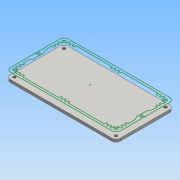
# Autodesk Inventor part: SZOMK-AK-C-C10-flat-plate
Saved by Autodesk Inventor 2016 (Build 200138000, 138)
## iProperties
Created: 2016-03-30
Part Number: SZOMK-AK-C-C10-flat-plate
Material: Generic
Document SubType Name: Modeling
Designer: admin
Density: 1 g/cm^3
Appearance: Default
Author: admin
Autodesk Inventor part; units mm, degrees
ref_plane "YZ Plane" through (0, 0, 0) normal (1, 0, 0) x (0, 1, 0)
ref_plane "XZ Plane" through (0, 0, 0) normal (0, 1, 0) x (-1, 0, 0)
ref_plane "XY Plane" through (0, 0, 0) normal (0, 0, 1) x (1, 0, 0)
derived "SZOMK-AK-C-C10-Walls.iam"
sketch "Sketch9" plane through (0, 0, 0) normal (0, 0, 1) x (1, 0, 0)
  line L0 (15.9674, 83.4048) -> (126.9674, 83.4048) projected
  arc A0 (15.9674, 83.4048) -> (11.4674, 78.9048) centre (15.9674, 78.9048) ccw projected
  line L1 (11.4674, 51.8798) -> (11.4674, 78.9048) projected
  line L2 (11.4674, 24.8548) -> (11.4674, 51.8798) projected
  arc A1 (11.4674, 24.8548) -> (15.9674, 20.3548) centre (15.9674, 24.8548) ccw projected
  line L3 (126.9674, 20.3548) -> (15.9674, 20.3548) projected
  arc A2 (126.9674, 20.3548) -> (131.4674, 24.8548) centre (126.9674, 24.8548) ccw projected
  line L4 (131.4674, 51.8798) -> (131.4674, 24.8548) projected
  line L5 (131.4674, 78.9048) -> (131.4674, 51.8798) projected
  arc A3 (131.4674, 78.9048) -> (126.9674, 83.4048) centre (126.9674, 78.9048) ccw projected
  point P0 (0, 0)
extrude "Extrusion3" add sketch "Sketch9" along normal blind 3
sketch "Sketch10" plane through (0, 0, 0) normal (0, 0, -1) x (-1, 0, 0)
  point P0 (0, 0)
  point P1 (-126.9674, 24.8548)
  point P2 (-126.9674, 78.9048)
  point P3 (-15.9674, 24.8548)
  point P4 (-15.9674, 78.9048)
hole "Hole1" at (126.9674, 78.9048, 0) at (126.9674, 24.8548, 0) at (15.9674, 24.8548, 0) at (15.9674, 78.9048, 0) direction (0, 0, 1) diameter 3 end through all countersink diameter 6 countersink angle 90
sketch "Sketch2" plane through (15.9674, 83.4048, 10) normal (0, 0, -1) x (1, 0, 0)
  line L0 (111, 31.525) -> (111, 24.3742) projected
  line L1 (111, 24.3742) -> (113, 21.6242) projected
  line L2 (113, 21.6242) -> (113, 15.7) projected
  line L3 (113, 15.7) -> (111, 15.7) projected
  line L4 (111, 15.7) -> (111, 13.7) projected
  line L5 (111, 13.7) -> (113, 13.7) projected
  line L6 (113, 13.7) -> (113, 11.7) projected
  line L7 (113, 11.7) -> (111, 11.7) projected
  line L8 (111, 11.7) -> (111, 9.7) projected
  line L9 (111, 9.7) -> (113, 9.7) projected
  line L10 (113, 9.7) -> (113, 7.3) projected
  line L11 (113, 7.3) -> (110.4678, 7.3) projected
  arc A0 (110.4678, 7.3) -> (110.1142, 6.4464) centre (110.4678, 6.8) ccw projected
  line L12 (110.1142, 6.4464) -> (110.6118, 5.9489) projected
  arc A1 (109.5511, 4.8882) -> (110.6118, 5.9489) centre (111, 4.5) ccw projected
  line L13 (109.5511, 4.8882) -> (109.0536, 5.3858) projected
  arc A2 (109.0536, 5.3858) -> (108.2, 5.0322) centre (108.7, 5.0322) ccw projected
  line L14 (108.2, 5.0322) -> (108.2, 2.3) projected
  line L15 (108.2, 2.3) -> (106.2, 2.3) projected
  line L16 (106.2, 2.3) -> (106.2, 4.5) projected
  line L17 (106.2, 4.5) -> (104.2, 4.5) projected
  line L18 (104.2, 4.5) -> (104.2, 2.3) projected
  line L19 (104.2, 2.3) -> (102.2, 2.3) projected
  line L20 (102.2, 2.3) -> (102.2, 4.5) projected
  line L21 (102.2, 4.5) -> (100.2, 4.5) projected
  line L22 (100.2, 4.5) -> (100.2, 2.3) projected
  line L23 (100.2, 2.3) -> (60.5, 2.3) projected
  line L24 (60.5, 2.3) -> (60.5, 4.5) projected
  line L25 (60.5, 4.5) -> (58.5, 4.5) projected
  line L26 (58.5, 4.5) -> (58.5, 2.3) projected
  line L27 (58.5, 2.3) -> (56.5, 2.3) projected
  line L28 (56.5, 2.3) -> (56.5, 4.5) projected
  line L29 (56.5, 4.5) -> (54.5, 4.5) projected
  line L30 (54.5, 4.5) -> (54.5, 2.3) projected
  line L31 (54.5, 2.3) -> (52.5, 2.3) projected
  line L32 (52.5, 2.3) -> (52.5, 4.5) projected
  line L33 (52.5, 4.5) -> (50.5, 4.5) projected
  line L34 (50.5, 4.5) -> (50.5, 2.3) projected
  line L35 (50.5, 2.3) -> (10.8, 2.3) projected
  line L36 (10.8, 2.3) -> (10.8, 4.5) projected
  line L37 (10.8, 4.5) -> (8.8, 4.5) projected
  line L38 (8.8, 4.5) -> (8.8, 2.3) projected
  line L39 (8.8, 2.3) -> (6.8, 2.3) projected
  line L40 (6.8, 2.3) -> (6.8, 4.5) projected
  line L41 (6.8, 4.5) -> (4.8, 4.5) projected
  line L42 (4.8, 4.5) -> (4.8, 2.3) projected
  line L43 (4.8, 2.3) -> (2.8, 2.3) projected
  line L44 (2.8, 2.3) -> (2.8, 5.0322) projected
  arc A3 (2.8, 5.0322) -> (1.9464, 5.3858) centre (2.3, 5.0322) ccw projected
  line L45 (1.9464, 5.3858) -> (1.4489, 4.8882) projected
  arc A4 (0.3882, 5.9489) -> (1.4489, 4.8882) centre (0, 4.5) ccw projected
  line L46 (0.3882, 5.9489) -> (0.8858, 6.4464) projected
  arc A5 (0.8858, 6.4464) -> (0.5322, 7.3) centre (0.5322, 6.8) ccw projected
  line L47 (0.5322, 7.3) -> (-2, 7.3) projected
  line L48 (-2, 7.3) -> (-2, 9.7) projected
  line L49 (-2, 9.7) -> (0, 9.7) projected
  line L50 (0, 9.7) -> (0, 11.7) projected
  line L51 (0, 11.7) -> (-2, 11.7) projected
  line L52 (-2, 11.7) -> (-2, 13.7) projected
  line L53 (-2, 13.7) -> (0, 13.7) projected
  line L54 (0, 13.7) -> (0, 15.7) projected
  line L55 (0, 15.7) -> (-2, 15.7) projected
  line L56 (-2, 15.7) -> (-2, 23.3362) projected
  line L57 (-2, 23.3362) -> (0, 26.7706) projected
  line L58 (0, 26.7706) -> (0, 31.525) projected
  line L59 (0, 31.525) -> (-1.5, 31.525) projected
  line L60 (-1.5, 31.525) -> (-1.5, 30.1864) projected
  arc A6 (-3, 30.1864) -> (-1.5, 30.1864) centre (-2.25, 29.525) ccw projected
  line L61 (-3, 30.1864) -> (-3, 31.525) projected
  line L62 (-3, 31.525) -> (-4.5, 31.525) projected
  line L63 (-4.5, 31.525) -> (-4.5, 4.5) projected
  arc A7 (-4.5, 4.5) -> (0, 0) centre (0, 4.5) ccw projected
  line L64 (0, 0) -> (111, 0) projected
  arc A8 (111, 0) -> (115.5, 4.5) centre (111, 4.5) ccw projected
  line L65 (115.5, 4.5) -> (115.5, 31.525) projected
  line L66 (115.5, 31.525) -> (114, 31.525) projected
  line L67 (114, 31.525) -> (114, 32.8636) projected
  arc A9 (114, 32.8636) -> (112.5, 32.8636) centre (113.25, 33.525) ccw projected
  line L68 (112.5, 32.8636) -> (112.5, 31.525) projected
  line L69 (112.5, 31.525) -> (111, 31.525) projected
  point P0 (55.5, 31.525)
sketch "Sketch2_1" plane through (15.9674, 20.3548, 10) normal (0, -1, 0) x (1, 0, 0)
  line L0 (44.2295, 1.8659) -> (36.146, 1.8659) construction
  line L1 (36.146, 1.8659) -> (36.146, 6.333) construction
  line L2 (36.146, 6.333) -> (44.2295, 6.333) construction
  line L3 (44.2295, 6.333) -> (44.2295, 1.8659) construction
  point P0 (55.5, 0)
sketch "Sketch3" plane through (126.9674, 20.3548, 10) normal (0, 0, -1) x (-1, 0, 0)
  line L0 (111, 31.525) -> (111, 24.3742) projected
  line L1 (111, 24.3742) -> (113, 21.6242) projected
  line L2 (113, 21.6242) -> (113, 15.7) projected
  line L3 (113, 15.7) -> (111, 15.7) projected
  line L4 (111, 15.7) -> (111, 13.7) projected
  line L5 (111, 13.7) -> (113, 13.7) projected
  line L6 (113, 13.7) -> (113, 11.7) projected
  line L7 (113, 11.7) -> (111, 11.7) projected
  line L8 (111, 11.7) -> (111, 9.7) projected
  line L9 (111, 9.7) -> (113, 9.7) projected
  line L10 (113, 9.7) -> (113, 7.3) projected
  line L11 (113, 7.3) -> (110.4678, 7.3) projected
  arc A0 (110.4678, 7.3) -> (110.1142, 6.4464) centre (110.4678, 6.8) ccw projected
  line L12 (110.1142, 6.4464) -> (110.6118, 5.9489) projected
  arc A1 (109.5511, 4.8882) -> (110.6118, 5.9489) centre (111, 4.5) ccw projected
  line L13 (109.5511, 4.8882) -> (109.0536, 5.3858) projected
  arc A2 (109.0536, 5.3858) -> (108.2, 5.0322) centre (108.7, 5.0322) ccw projected
  line L14 (108.2, 5.0322) -> (108.2, 2.3) projected
  line L15 (108.2, 2.3) -> (106.2, 2.3) projected
  line L16 (106.2, 2.3) -> (106.2, 4.5) projected
  line L17 (106.2, 4.5) -> (104.2, 4.5) projected
  line L18 (104.2, 4.5) -> (104.2, 2.3) projected
  line L19 (104.2, 2.3) -> (102.2, 2.3) projected
  line L20 (102.2, 2.3) -> (102.2, 4.5) projected
  line L21 (102.2, 4.5) -> (100.2, 4.5) projected
  line L22 (100.2, 4.5) -> (100.2, 2.3) projected
  line L23 (100.2, 2.3) -> (60.5, 2.3) projected
  line L24 (60.5, 2.3) -> (60.5, 4.5) projected
  line L25 (60.5, 4.5) -> (58.5, 4.5) projected
  line L26 (58.5, 4.5) -> (58.5, 2.3) projected
  line L27 (58.5, 2.3) -> (56.5, 2.3) projected
  line L28 (56.5, 2.3) -> (56.5, 4.5) projected
  line L29 (56.5, 4.5) -> (54.5, 4.5) projected
  line L30 (54.5, 4.5) -> (54.5, 2.3) projected
  line L31 (54.5, 2.3) -> (52.5, 2.3) projected
  line L32 (52.5, 2.3) -> (52.5, 4.5) projected
  line L33 (52.5, 4.5) -> (50.5, 4.5) projected
  line L34 (50.5, 4.5) -> (50.5, 2.3) projected
  line L35 (50.5, 2.3) -> (10.8, 2.3) projected
  line L36 (10.8, 2.3) -> (10.8, 4.5) projected
  line L37 (10.8, 4.5) -> (8.8, 4.5) projected
  line L38 (8.8, 4.5) -> (8.8, 2.3) projected
  line L39 (8.8, 2.3) -> (6.8, 2.3) projected
  line L40 (6.8, 2.3) -> (6.8, 4.5) projected
  line L41 (6.8, 4.5) -> (4.8, 4.5) projected
  line L42 (4.8, 4.5) -> (4.8, 2.3) projected
  line L43 (4.8, 2.3) -> (2.8, 2.3) projected
  line L44 (2.8, 2.3) -> (2.8, 5.0322) projected
  arc A3 (2.8, 5.0322) -> (1.9464, 5.3858) centre (2.3, 5.0322) ccw projected
  line L45 (1.9464, 5.3858) -> (1.4489, 4.8882) projected
  arc A4 (0.3882, 5.9489) -> (1.4489, 4.8882) centre (0, 4.5) ccw projected
  line L46 (0.3882, 5.9489) -> (0.8858, 6.4464) projected
  arc A5 (0.8858, 6.4464) -> (0.5322, 7.3) centre (0.5322, 6.8) ccw projected
  line L47 (0.5322, 7.3) -> (-2, 7.3) projected
  line L48 (-2, 7.3) -> (-2, 9.7) projected
  line L49 (-2, 9.7) -> (0, 9.7) projected
  line L50 (0, 9.7) -> (0, 11.7) projected
  line L51 (0, 11.7) -> (-2, 11.7) projected
  line L52 (-2, 11.7) -> (-2, 13.7) projected
  line L53 (-2, 13.7) -> (0, 13.7) projected
  line L54 (0, 13.7) -> (0, 15.7) projected
  line L55 (0, 15.7) -> (-2, 15.7) projected
  line L56 (-2, 15.7) -> (-2, 23.3362) projected
  line L57 (-2, 23.3362) -> (0, 26.7706) projected
  line L58 (0, 26.7706) -> (0, 31.525) projected
  line L59 (0, 31.525) -> (-1.5, 31.525) projected
  line L60 (-1.5, 31.525) -> (-1.5, 30.1864) projected
  arc A6 (-3, 30.1864) -> (-1.5, 30.1864) centre (-2.25, 29.525) ccw projected
  line L61 (-3, 30.1864) -> (-3, 31.525) projected
  line L62 (-3, 31.525) -> (-4.5, 31.525) projected
  line L63 (-4.5, 31.525) -> (-4.5, 4.5) projected
  arc A7 (-4.5, 4.5) -> (0, 0) centre (0, 4.5) ccw projected
  line L64 (0, 0) -> (111, 0) projected
  arc A8 (111, 0) -> (115.5, 4.5) centre (111, 4.5) ccw projected
  line L65 (115.5, 4.5) -> (115.5, 31.525) projected
  line L66 (115.5, 31.525) -> (114, 31.525) projected
  line L67 (114, 31.525) -> (114, 32.8636) projected
  arc A9 (114, 32.8636) -> (112.5, 32.8636) centre (113.25, 33.525) ccw projected
  line L68 (112.5, 32.8636) -> (112.5, 31.525) projected
  line L69 (112.5, 31.525) -> (111, 31.525) projected
  point P0 (55.5, 31.525)
body "Solid6"
